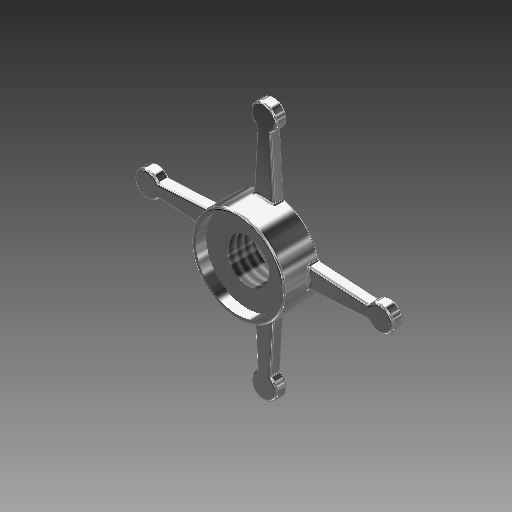
# Autodesk Inventor part: 308-04
Saved by Autodesk Inventor 2019 (Build 230136000, 136)
## iProperties
Company: Autodesk Inc.
Created: 2012-01-25
Part Number: 308-04
Material: Aluminum-6061
Document SubType Name: Modeling
Designer: Autodesk Inc.
Mass: 4.49689 g
Surface Area: 17.1265 cm^2
Volume: 1.66552 cm^3
Density: 2.7 g/cm^3
Appearance: Chrome - Polished
Author: Inventor
Autodesk Inventor part; units mm, degrees
ref_plane "YZ Plane" through (0, 0, 0) normal (1, 0, 0) x (0, 1, 0)
ref_plane "XZ Plane" through (0, 0, 0) normal (0, 1, 0) x (-1, 0, 0)
ref_plane "XY Plane" through (0, 0, 0) normal (0, 0, 1) x (1, 0, 0)
sketch "Sketch1" plane through (0, 0, 0) normal (0, 0, 1) x (1, 0, 0)
  line L0 (0, 0) -> (6.364, 6.364)
  line L1 (0, 0) -> (9, 0) construction
  arc A0 (6.364, -6.364) -> (6.364, 6.364) centre (0, 0) ccw
  line L2 (6.364, -6.364) -> (0, 0)
  line L3 (8.775, 2) -> (8.775, -2) construction
  line L4 (9, 0) -> (22.5, 0) construction
  circle A1 centre (22.5, 0) radius 2.5
  line L5 (20.3646, 1.3) -> (20.3646, -1.3) construction
  line L6 (8.775, 2) -> (20.3646, 1.3)
  line L7 (20.3646, -1.3) -> (8.775, -2)
  dimension "d0" = 9
  dimension "d1" = 45
  dimension "d2" = 4
  dimension "d3" = 22.5
  dimension "d4" = 5
  dimension "d5" = 2.6
  constraints: 16 end point, 6 point on circle, 4 perpendicular, 2 centre point, 2 equal length, 1 coincident, 1 horizontal, 1 point on line
  measures "d0" distance of L0.start L0.end
  measures "d1" angle of L1 L0
  measures "d2" distance of L3.start L3.end
  measures "d3" distance of L0.start L4.end
  measures "d4" diameter of A1
  measures "d5" distance of L5.start L5.end
extrude "Extrusion1" add sketch "Sketch1" along normal blind 2.3
extrude "Extrusion2" add sketch "Sketch1" along normal blind 7.3 contours L0 A0 L2
fillet "Fillet1" radius 0.5 14 edges at (8.775, -2, 1.15) (8.775, 2, 1.15) (20.3646, -1.3, 1.15) (20.3646, 1.3, 1.15) (14.5698, -1.65, 2.3) (25, 0, 2.3) (14.5698, 1.65, 2.3) (7.8777, -4.3523, 0) (9, 0, 7.3) (7.8777, 4.3523, 0) (14.5698, 1.65, 0) (25, 0, 0) (14.5698, -1.65, 0) (9, 0, 2.3)
pattern_circular "Circular Pattern1" count 4 over 360 about axis through (0, 0, 0) along (0, 0, 1)
hole "Hole1" at (0, 0, 7.3) direction (0, 0, -1) diameter 8.376 end through all counterbore diameter 16 counterbore depth 2 thread size "M10x1.5" class "6H" standard "ANSI Metric M Profile"
body "Solid1"
